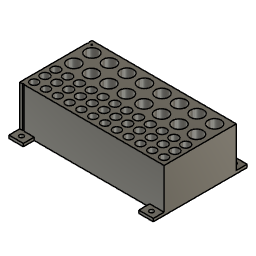
vial rack v6 (Autodesk Fusion 360 design; units mm, degrees)
Autodesk Fusion 360 part; units mm, degrees
sketch "Sketch2" plane through (0, 0, 0) normal (0, 0, 1) x (1, 0, 0)
  line L0 (0, 0) -> (200, 0)
  line L1 (200, 0) -> (200, 100)
  line L2 (200, 100) -> (0, 100)
  line L3 (0, 100) -> (0, 0)
  dimension "d31" = 200
  dimension "d32" = 100
  constraint horizontal L0
  constraint vertical L1
  constraint horizontal L2
  constraint vertical L3
  constraint coincident L0.start L3.end
  measures "d31" distance of L0.start L0.end
  measures "d32" distance of L0.start L2.end
extrude "Extrude2" add sketch "Sketch2" along normal blind 60
sketch "Sketch3" plane through (0, 0, 60) normal (0, 0, 1) x (-1, 0, 0)
  line L0 (0, -100) -> (0, 0)
  line L1 (0, 0) -> (-200, 0)
  line L2 (-200, 0) -> (-200, -100)
  line L3 (-200, -100) -> (0, -100)
  circle A0 centre (-15, -85) radius 9
  circle A1 centre (-39.2857, -85) radius 9
  circle A2 centre (-63.5714, -85) radius 9
  circle A3 centre (-87.8571, -85) radius 9
  circle A4 centre (-112.1429, -85) radius 9
  circle A5 centre (-136.4286, -85) radius 9
  circle A6 centre (-160.7143, -85) radius 9
  circle A7 centre (-185, -85) radius 9
  circle A8 centre (-15, -60) radius 9
  circle A9 centre (-39.2857, -60) radius 9
  circle A10 centre (-63.5714, -60) radius 9
  circle A11 centre (-87.8571, -60) radius 9
  circle A12 centre (-112.1429, -60) radius 9
  circle A13 centre (-136.4286, -60) radius 9
  circle A14 centre (-160.7143, -60) radius 9
  circle A15 centre (-185, -60) radius 9
  dimension "d35" = 18
  dimension "d36" = 15
  dimension "d37" = 15
  dimension "d40" = -170
  dimension "d41" = 0
  dimension "d44" = 0
  dimension "d45" = 25
  measures "d35" diameter of A0
  measures "d36" distance of L3 A0.centre
  measures "d37" distance of L0 A0.centre
extrude "Extrude3" cut sketch "Sketch3" against normal blind 30 contours A0 | A1 | A2 | A3 | A4 | A5 | A6 | A7 | A8 | A9 | A10 | A11 | A12 | A13 | A14 | A15
sketch "Sketch4" plane through (0, 0, 60) normal (0, 0, 1) x (-1, 0, 0)
  circle A0 centre (-63.5714, -60) radius 9
  circle A1 centre (-160.7143, -60) radius 9
  circle A2 centre (-136.4286, -85) radius 9
  circle A3 centre (-39.2857, -85) radius 9
  circle A4 centre (-63.5714, -85) radius 9
  circle A5 centre (-160.7143, -85) radius 9
  circle A6 centre (-136.4286, -60) radius 9
  circle A7 centre (-39.2857, -60) radius 9
  circle A8 centre (-87.8571, -60) radius 9
  circle A9 centre (-185, -60) radius 9
  circle A10 centre (-112.1429, -85) radius 9
  circle A11 centre (-15, -85) radius 9
  circle A12 centre (-87.8571, -85) radius 9
  circle A13 centre (-185, -85) radius 9
  circle A14 centre (-112.1429, -60) radius 9
  circle A15 centre (-15, -60) radius 9
  line L0 (0, -100) -> (0, 0)
  line L1 (0, 0) -> (-200, 0)
  line L2 (-200, 0) -> (-200, -100)
  line L3 (-200, -100) -> (0, -100)
  circle A16 centre (-10, -40) radius 6
  circle A17 centre (-26.3636, -40) radius 6
  circle A18 centre (-42.7273, -40) radius 6
  circle A19 centre (-59.0909, -40) radius 6
  circle A20 centre (-75.4545, -40) radius 6
  circle A21 centre (-91.8182, -40) radius 6
  circle A22 centre (-108.1818, -40) radius 6
  circle A23 centre (-124.5455, -40) radius 6
  circle A24 centre (-140.9091, -40) radius 6
  circle A25 centre (-157.2727, -40) radius 6
  circle A26 centre (-173.6364, -40) radius 6
  circle A27 centre (-190, -40) radius 6
  circle A28 centre (-10, -25) radius 6
  circle A29 centre (-26.3636, -25) radius 6
  circle A30 centre (-42.7273, -25) radius 6
  circle A31 centre (-59.0909, -25) radius 6
  circle A32 centre (-75.4545, -25) radius 6
  circle A33 centre (-91.8182, -25) radius 6
  circle A34 centre (-108.1818, -25) radius 6
  circle A35 centre (-124.5455, -25) radius 6
  circle A36 centre (-140.9091, -25) radius 6
  circle A37 centre (-157.2727, -25) radius 6
  circle A38 centre (-173.6364, -25) radius 6
  circle A39 centre (-190, -25) radius 6
  circle A40 centre (-10, -10) radius 5.5
  circle A41 centre (-26.3636, -10) radius 5.5
  circle A42 centre (-42.7273, -10) radius 5.5
  circle A43 centre (-59.0909, -10) radius 5.5
  circle A44 centre (-75.4545, -10) radius 5.5
  circle A45 centre (-91.8182, -10) radius 5.5
  circle A46 centre (-108.1818, -10) radius 5.5
  circle A47 centre (-124.5455, -10) radius 5.5
  circle A48 centre (-140.9091, -10) radius 5.5
  circle A49 centre (-157.2727, -10) radius 5.5
  circle A50 centre (-173.6364, -10) radius 5.5
  circle A51 centre (-190, -10) radius 5.5
  dimension "d48" = 12
  dimension "d49" = 10
  dimension "d52" = -180
  dimension "d53" = 0
  dimension "d56" = 0
  dimension "d57" = 15
  dimension "d58" = 11
  dimension "d61" = -180
  dimension "d62" = 0
  measures "d48" diameter of A16
  measures "d49" distance of L0 A16.centre
  measures "d58" diameter of A40
extrude "Extrude4" cut sketch "Sketch4" against normal blind 20 contours A16 | A17 | A18 | A19 | A20 | A21 | A22 | A23 | A24 | A25 | A26 | A27 | A28 | A29 | A30 | A31 | A32 | A33 | A34 | A35 | A36 | A37 | A38 | A39
sketch "Sketch5" plane through (0, 0, 60) normal (0, 0, 1) x (-1, 0, 0)
  circle A0 centre (-42.7273, -25) radius 6
  circle A1 centre (-108.1818, -25) radius 6
  circle A2 centre (-173.6364, -25) radius 6
  circle A3 centre (-157.2727, -40) radius 6
  circle A4 centre (-91.8182, -40) radius 6
  circle A5 centre (-26.3636, -40) radius 6
  circle A6 centre (-42.7273, -40) radius 6
  circle A7 centre (-108.1818, -40) radius 6
  circle A8 centre (-173.6364, -40) radius 6
  circle A9 centre (-157.2727, -25) radius 6
  circle A10 centre (-91.8182, -25) radius 6
  circle A11 centre (-26.3636, -25) radius 6
  circle A12 centre (-59.0909, -25) radius 6
  circle A13 centre (-124.5455, -25) radius 6
  circle A14 centre (-190, -25) radius 6
  circle A15 centre (-140.9091, -40) radius 6
  circle A16 centre (-75.4545, -40) radius 6
  circle A17 centre (-10, -40) radius 6
  circle A18 centre (-59.0909, -40) radius 6
  circle A19 centre (-124.5455, -40) radius 6
  circle A20 centre (-190, -40) radius 6
  circle A21 centre (-140.9091, -25) radius 6
  circle A22 centre (-75.4545, -25) radius 6
  circle A23 centre (-10, -25) radius 6
  circle A24 centre (-63.5714, -60) radius 9
  circle A25 centre (-160.7143, -60) radius 9
  circle A26 centre (-136.4286, -85) radius 9
  circle A27 centre (-39.2857, -85) radius 9
  circle A28 centre (-63.5714, -85) radius 9
  circle A29 centre (-160.7143, -85) radius 9
  circle A30 centre (-136.4286, -60) radius 9
  circle A31 centre (-39.2857, -60) radius 9
  circle A32 centre (-87.8571, -60) radius 9
  circle A33 centre (-185, -60) radius 9
  circle A34 centre (-112.1429, -85) radius 9
  circle A35 centre (-15, -85) radius 9
  circle A36 centre (-87.8571, -85) radius 9
  circle A37 centre (-185, -85) radius 9
  circle A38 centre (-112.1429, -60) radius 9
  circle A39 centre (-15, -60) radius 9
  line L0 (0, -100) -> (0, 0)
  line L1 (0, 0) -> (-200, 0)
  line L2 (-200, 0) -> (-200, -100)
  line L3 (-200, -100) -> (0, -100)
  circle A40 centre (-10, -10) radius 5.5
  circle A41 centre (-26.3636, -10) radius 5.5
  circle A42 centre (-42.7273, -10) radius 5.5
  circle A43 centre (-59.0909, -10) radius 5.5
  circle A44 centre (-75.4545, -10) radius 5.5
  circle A45 centre (-91.8182, -10) radius 5.5
  circle A46 centre (-108.1818, -10) radius 5.5
  circle A47 centre (-124.5455, -10) radius 5.5
  circle A48 centre (-140.9091, -10) radius 5.5
  circle A49 centre (-157.2727, -10) radius 5.5
  circle A50 centre (-173.6364, -10) radius 5.5
  circle A51 centre (-190, -10) radius 5.5
  dimension "d65" = 11
  dimension "d68" = -180
  dimension "d69" = 0
  measures "d65" diameter of A40
extrude "Extrude5" cut sketch "Sketch5" against normal blind 30 contours A40 | A41 | A42 | A43 | A44 | A45 | A46 | A47 | A48 | A49 | A50 | A51
sketch "Sketch6" plane through (0, 0, 0) normal (0, -1, 0) x (1, 0, 0)
  line L0 (0, 0) -> (200, 0)
  line L1 (200, 0) -> (200, 60)
  line L2 (200, 60) -> (0, 60)
  line L3 (0, 60) -> (0, 0)
  line L4 (0, 0) -> (20, 0)
  line L5 (20, 0) -> (20, 4)
  line L6 (20, 4) -> (0, 4)
  line L7 (0, 4) -> (0, 0)
  line L8 (200, 0) -> (180, 0)
  line L9 (180, 0) -> (180, 4)
  line L10 (180, 4) -> (200, 4)
  line L11 (200, 4) -> (200, 0)
  dimension "d72" = 20
  dimension "d73" = 4
  dimension "d74" = 20
  dimension "d75" = 4
  constraint horizontal L4
  constraint vertical L5
  constraint horizontal L6
  constraint vertical L7
  constraint coincident L0.start L3.end
  constraint horizontal L8
  constraint vertical L9
  constraint horizontal L10
  constraint vertical L11
  constraint coincident L0.end L1.start
  measures "d72" distance of L0.start L4.end
  measures "d73" distance of L0.start L6.end
  measures "d74" distance of L0.end L8.end
  measures "d75" distance of L0.end L10.end
extrude "Extrude6" add sketch "Sketch6" along normal blind 15 contours L0 L3 L4 L5 L6 L7 | L0 L1 L8 L9 L10 L11
sketch "Sketch7" plane through (0, 100, 0) normal (0, 1, 0) x (-1, 0, 0)
  line L0 (-200, 0) -> (0, 0)
  line L1 (0, 0) -> (0, 60)
  line L2 (0, 60) -> (-200, 60)
  line L3 (-200, 60) -> (-200, 0)
  line L4 (-200, 0) -> (-180, 0)
  line L5 (-180, 0) -> (-180, 4)
  line L6 (-180, 4) -> (-200, 4)
  line L7 (-200, 4) -> (-200, 0)
  line L8 (0, 0) -> (-20, 0)
  line L9 (-20, 0) -> (-20, 4)
  line L10 (-20, 4) -> (0, 4)
  line L11 (0, 4) -> (0, 0)
  dimension "d78" = 20
  dimension "d79" = 4
  dimension "d80" = 20
  dimension "d81" = 4
  constraint horizontal L4
  constraint vertical L5
  constraint horizontal L6
  constraint vertical L7
  constraint coincident L0.start L3.end
  constraint horizontal L8
  constraint vertical L9
  constraint horizontal L10
  constraint vertical L11
  constraint coincident L0.end L1.start
  measures "d78" distance of L0.start L4.end
  measures "d79" distance of L0.start L6.end
  measures "d80" distance of L0.end L8.end
  measures "d81" distance of L0.end L10.end
extrude "Extrude7" add sketch "Sketch7" along normal blind 15 contours L0 L3 L4 L5 L6 L7 | L0 L1 L8 L9 L10 L11
sketch "Sketch8" plane through (0, 0, 4) normal (0, 0, 1) x (-1, 0, 0)
  line L0 (-180, -100) -> (-200, -100)
  line L1 (-200, -100) -> (-200, -115)
  line L2 (-200, -115) -> (-180, -115)
  line L3 (-180, -115) -> (-180, -100)
  circle A0 centre (-190, -107.5) radius 3
  dimension "d84" = 6
  dimension "d85" = 10
  dimension "d86" = 7.5
  measures "d84" diameter of A0
  measures "d85" distance of L1 A0.centre
  measures "d86" distance of L2 A0.centre
extrude "Extrude8" cut sketch "Sketch8" against normal blind 4 contours A0
sketch "Sketch9" plane through (0, 0, 4) normal (0, 0, 1) x (-1, 0, 0)
  line L0 (-200, 0) -> (-180, 0)
  line L1 (-180, 0) -> (-180, 15)
  line L2 (-180, 15) -> (-200, 15)
  line L3 (-200, 15) -> (-200, 0)
  circle A0 centre (-190, 7.5) radius 3
  dimension "d89" = 6
  dimension "d90" = 7.5
  dimension "d91" = 10
  measures "d89" diameter of A0
  measures "d90" distance of L2 A0.centre
  measures "d91" distance of L3 A0.centre
extrude "Extrude9" cut sketch "Sketch9" against normal blind 4 contours A0
sketch "Sketch10" plane through (0, 0, 4) normal (0, 0, 1) x (-1, 0, 0)
  line L0 (-20, 0) -> (0, 0)
  line L1 (0, 0) -> (0, 15)
  line L2 (0, 15) -> (-20, 15)
  line L3 (-20, 15) -> (-20, 0)
  circle A0 centre (-10, 7.5) radius 3
  dimension "d94" = 6
  dimension "d95" = 7.5
  dimension "d96" = 10
  measures "d94" diameter of A0
  measures "d95" distance of L2 A0.centre
  measures "d96" distance of L3 A0.centre
extrude "Extrude10" cut sketch "Sketch10" against normal blind 4 contours A0
sketch "Sketch11" plane through (0, 0, 4) normal (0, 0, 1) x (-1, 0, 0)
  line L0 (0, -100) -> (-20, -100)
  line L1 (-20, -100) -> (-20, -115)
  line L2 (-20, -115) -> (0, -115)
  line L3 (0, -115) -> (0, -100)
  circle A0 centre (-10, -107.5) radius 3
  dimension "d99" = 6
  dimension "d100" = 7.5
  dimension "d101" = 10
  measures "d99" diameter of A0
  measures "d100" distance of L2 A0.centre
  measures "d101" distance of L1 A0.centre
extrude "Extrude11" cut sketch "Sketch11" against normal blind 4 contours A0
sketch "Sketch12" plane through (0, 0, 60) normal (0, 0, 1) x (-1, 0, 0)
  circle A0 centre (-157.2727, -10) radius 5.5
  circle A1 centre (-91.8182, -10) radius 5.5
  circle A2 centre (-26.3636, -10) radius 5.5
  circle A3 centre (-42.7273, -10) radius 5.5
  circle A4 centre (-108.1818, -10) radius 5.5
  circle A5 centre (-173.6364, -10) radius 5.5
  circle A6 centre (-140.9091, -10) radius 5.5
  circle A7 centre (-75.4545, -10) radius 5.5
  circle A8 centre (-10, -10) radius 5.5
  circle A9 centre (-59.0909, -10) radius 5.5
  circle A10 centre (-124.5455, -10) radius 5.5
  circle A11 centre (-190, -10) radius 5.5
  circle A12 centre (-42.7273, -25) radius 6
  circle A13 centre (-108.1818, -25) radius 6
  circle A14 centre (-173.6364, -25) radius 6
  circle A15 centre (-157.2727, -40) radius 6
  circle A16 centre (-91.8182, -40) radius 6
  circle A17 centre (-26.3636, -40) radius 6
  circle A18 centre (-42.7273, -40) radius 6
  circle A19 centre (-108.1818, -40) radius 6
  circle A20 centre (-173.6364, -40) radius 6
  circle A21 centre (-157.2727, -25) radius 6
  circle A22 centre (-91.8182, -25) radius 6
  circle A23 centre (-26.3636, -25) radius 6
  circle A24 centre (-59.0909, -25) radius 6
  circle A25 centre (-124.5455, -25) radius 6
  circle A26 centre (-190, -25) radius 6
  circle A27 centre (-140.9091, -40) radius 6
  circle A28 centre (-75.4545, -40) radius 6
  circle A29 centre (-10, -40) radius 6
  circle A30 centre (-59.0909, -40) radius 6
  circle A31 centre (-124.5455, -40) radius 6
  circle A32 centre (-190, -40) radius 6
  circle A33 centre (-140.9091, -25) radius 6
  circle A34 centre (-75.4545, -25) radius 6
  circle A35 centre (-10, -25) radius 6
  circle A36 centre (-63.5714, -60) radius 9
  circle A37 centre (-160.7143, -60) radius 9
  circle A38 centre (-136.4286, -85) radius 9
  circle A39 centre (-39.2857, -85) radius 9
  circle A40 centre (-63.5714, -85) radius 9
  circle A41 centre (-160.7143, -85) radius 9
  circle A42 centre (-136.4286, -60) radius 9
  circle A43 centre (-39.2857, -60) radius 9
  circle A44 centre (-87.8571, -60) radius 9
  circle A45 centre (-185, -60) radius 9
  circle A46 centre (-112.1429, -85) radius 9
  circle A47 centre (-15, -85) radius 9
  circle A48 centre (-87.8571, -85) radius 9
  circle A49 centre (-185, -85) radius 9
  circle A50 centre (-112.1429, -60) radius 9
  circle A51 centre (-15, -60) radius 9
  line L0 (0, -100) -> (0, 0)
  line L1 (0, 0) -> (-200, 0)
  line L2 (-200, 0) -> (-200, -100)
  line L3 (-200, -100) -> (0, -100)
  circle A52 centre (-5, -95) radius 1
extrude "Extrude12" cut sketch "Sketch12" against normal blind 30 contours A52
sketch "Sketch13" plane through (0, 0, 60) normal (0, 0, 1) x (-1, 0, 0)
  circle A0 centre (-5, -95) radius 1
  circle A1 centre (-157.2727, -10) radius 5.5
  circle A2 centre (-91.8182, -10) radius 5.5
  circle A3 centre (-26.3636, -10) radius 5.5
  circle A4 centre (-42.7273, -10) radius 5.5
  circle A5 centre (-108.1818, -10) radius 5.5
  circle A6 centre (-173.6364, -10) radius 5.5
  circle A7 centre (-140.9091, -10) radius 5.5
  circle A8 centre (-75.4545, -10) radius 5.5
  circle A9 centre (-10, -10) radius 5.5
  circle A10 centre (-59.0909, -10) radius 5.5
  circle A11 centre (-124.5455, -10) radius 5.5
  circle A12 centre (-190, -10) radius 5.5
  circle A13 centre (-42.7273, -25) radius 6
  circle A14 centre (-108.1818, -25) radius 6
  circle A15 centre (-173.6364, -25) radius 6
  circle A16 centre (-157.2727, -40) radius 6
  circle A17 centre (-91.8182, -40) radius 6
  circle A18 centre (-26.3636, -40) radius 6
  circle A19 centre (-42.7273, -40) radius 6
  circle A20 centre (-108.1818, -40) radius 6
  circle A21 centre (-173.6364, -40) radius 6
  circle A22 centre (-157.2727, -25) radius 6
  circle A23 centre (-91.8182, -25) radius 6
  circle A24 centre (-26.3636, -25) radius 6
  circle A25 centre (-59.0909, -25) radius 6
  circle A26 centre (-124.5455, -25) radius 6
  circle A27 centre (-190, -25) radius 6
  circle A28 centre (-140.9091, -40) radius 6
  circle A29 centre (-75.4545, -40) radius 6
  circle A30 centre (-10, -40) radius 6
  circle A31 centre (-59.0909, -40) radius 6
  circle A32 centre (-124.5455, -40) radius 6
  circle A33 centre (-190, -40) radius 6
  circle A34 centre (-140.9091, -25) radius 6
  circle A35 centre (-75.4545, -25) radius 6
  circle A36 centre (-10, -25) radius 6
  circle A37 centre (-63.5714, -60) radius 9
  circle A38 centre (-160.7143, -60) radius 9
  circle A39 centre (-136.4286, -85) radius 9
  circle A40 centre (-39.2857, -85) radius 9
  circle A41 centre (-63.5714, -85) radius 9
  circle A42 centre (-160.7143, -85) radius 9
  circle A43 centre (-136.4286, -60) radius 9
  circle A44 centre (-39.2857, -60) radius 9
  circle A45 centre (-87.8571, -60) radius 9
  circle A46 centre (-185, -60) radius 9
  circle A47 centre (-112.1429, -85) radius 9
  circle A48 centre (-15, -85) radius 9
  circle A49 centre (-87.8571, -85) radius 9
  circle A50 centre (-185, -85) radius 9
  circle A51 centre (-112.1429, -60) radius 9
  circle A52 centre (-15, -60) radius 9
  line L0 (0, -100) -> (0, 0)
  line L1 (0, 0) -> (-200, 0)
  line L2 (-200, 0) -> (-200, -100)
  line L3 (-200, -100) -> (0, -100)
  circle A53 centre (0, -95) radius 1
  circle A54 centre (-5, 0) radius 1
  constraint coincident L0 A53.centre
  constraint coincident L1 A54.centre
extrude "Extrude13" cut sketch "Sketch13" against normal blind 56 contours L0 A53 | L1 A54 picked at (-0.2606, -94.7922) picked at (-5.2041, -0.3103)
